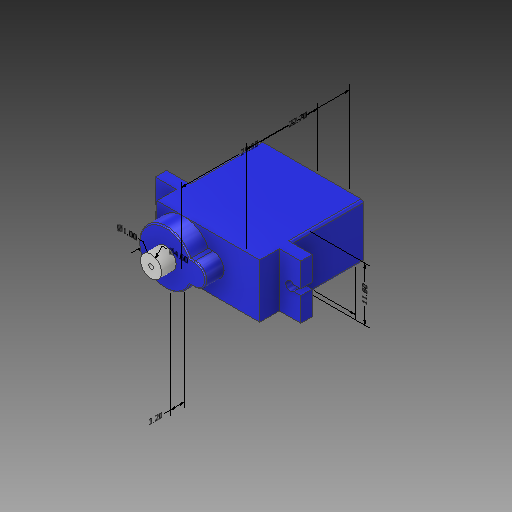
# Autodesk Inventor part: servo motor
Saved by Autodesk Inventor 2018 (Build 220112000, 112)
## iProperties
Created: 2017-05-17
Part Number: servo motor
Material: Generic
Document SubType Name: Modeling
Designer: Manh
Density: 1 g/cm^3
Appearance: Default
Author: Manh
Autodesk Inventor part; units mm, degrees
ref_plane "YZ Plane" through (0, 0, 0) normal (1, 0, 0) x (0, 1, 0)
ref_plane "XZ Plane" through (0, 0, 0) normal (0, 1, 0) x (-1, 0, 0)
ref_plane "XY Plane" through (0, 0, 0) normal (0, 0, 1) x (1, 0, 0)
sketch "Sketch1" plane through (0, 0, 0) normal (0, 0, 1) x (1, 0, 0)
  line L0 (-11.5182, 8.1773) -> (10.9818, 8.1773)
  line L1 (10.9818, 8.1773) -> (10.9818, -3.6227)
  line L2 (10.9818, -3.6227) -> (-11.5182, -3.6227)
  line L3 (-11.5182, -3.6227) -> (-11.5182, 8.1773)
  point P0 (0, 0)
  dimension "d0" = 22.5
  dimension "d1" = 11.8
  constraints: 8 end point, 2 parallel, 1 horizontal, 1 perpendicular
  measures "d0" distance of L1.end L2.end
  measures "d1" distance of L0.end L1.end
extrude "Extrusion1" add sketch "Sketch1" along normal blind 22.7
sketch "Sketch2" plane through (0, 0, 22.7) normal (0, 0, 1) x (1, 0, 0)
  arc A0 (-0.2741, 4.7773) -> (-0.2741, -0.2227) centre (-5.6182, 2.2773) ccw
  line L0 (-11.5182, 8.1773) -> (-11.5182, -3.6227) projected
  line L1 (-11.5182, -3.6227) -> (10.9818, -3.6227) projected
  line L2 (-0.2741, 4.7773) -> (0.6818, 4.7773)
  line L3 (0.6818, -0.2227) -> (-0.2741, -0.2227)
  arc A1 (0.6818, -0.2227) -> (0.6818, 4.7773) centre (0.6818, 2.2773) ccw
  line L4 (3.1818, 2.2773) -> (3.1818, 4.4746) construction
  point P0 (0, 0)
  dimension "d4" = 11.8
  dimension "d5" = 5.9
  dimension "d6" = 5
  dimension "d7" = 8.8
  dimension "d8" = 2.5
  constraints: 6 end point, 5 point on circle, 4 tangent, 2 centre point, 2 horizontal, 1 horizontal alignment, 1 vertical
  measures "d4" diameter of A0
  measures "d5" distance from line of L1 A0.centre
  measures "d6" distance of L2.end L3.start
  measures "d7" distance from line of A0.centre L4
  measures "d8" radius of A1
extrude "Extrusion2" add sketch "Sketch2" along normal blind 4 contours L2 A1 L3 A0
sketch "Sketch3" plane through (0, 0, 26.7) normal (0, 0, 1) x (1, 0, 0)
  line L0 (0.6818, 4.7773) -> (-0.2741, 4.7773) projected
  arc A0 (-0.2741, 4.7773) -> (-0.2741, -0.2227) centre (-5.6182, 2.2773) ccw projected
  line L1 (-0.2741, -0.2227) -> (0.6818, -0.2227) projected
  arc A1 (0.6818, -0.2227) -> (0.6818, 4.7773) centre (0.6818, 2.2773) ccw projected
  circle A2 centre (-5.6182, 2.2773) radius 2.3
  point P0 (0, 0)
  dimension "d11" = 4.6
  constraints: 1 centre point, 1 coincident
  measures "d11" diameter of A2
extrude "Extrusion3" add sketch "Sketch3" along normal blind 3.2 contours A2
ref_plane "Work Plane1" through (0, 0, 18.4) normal (0, 0, -1) x (-1, 0, 0)
sketch "Sketch4" plane through (0, 0, 18.4) normal (0, 0, -1) x (-1, 0, 0)
  line L0 (11.5182, 8.1773) -> (-10.9818, 8.1773) projected
  line L1 (-10.9818, 8.1773) -> (-10.9818, -3.6227) projected
  line L2 (-10.9818, -3.6227) -> (11.5182, -3.6227) projected
  line L3 (11.5182, -3.6227) -> (11.5182, 8.1773) projected
  line L4 (11.5182, 8.1773) -> (16.2182, 8.1773)
  line L5 (16.2182, 8.1773) -> (16.2182, -3.6227)
  line L6 (16.2182, -3.6227) -> (11.5182, -3.6227)
  line L7 (11.5182, -3.6227) -> (11.5182, 8.1773)
  line L8 (-10.9818, 8.1773) -> (-15.6818, 8.1773)
  line L9 (-15.6818, 8.1773) -> (-15.6818, -3.6227)
  line L10 (-15.6818, -3.6227) -> (-10.9818, -3.6227)
  line L11 (-10.9818, -3.6227) -> (-10.9818, 8.1773)
  arc A0 (14.6782, 2.9273) -> (14.6782, 1.6273) centre (13.9182, 2.2773) ccw
  arc A1 (-14.1417, 1.6273) -> (-14.1417, 2.9273) centre (-13.3818, 2.2773) ccw
  line L12 (-14.1417, 2.9273) -> (-15.6818, 2.9273)
  line L13 (-14.1417, 1.6273) -> (-15.6818, 1.6273)
  line L14 (16.2182, 2.9273) -> (14.6782, 2.9273)
  line L15 (16.2182, 1.6273) -> (14.6782, 1.6273)
  point P0 (0, 0)
  dimension "d15" = 4.7
  dimension "d16" = 4.7
  dimension "d17" = 5.9
  dimension "d18" = 5.9
  dimension "d19" = 2
  dimension "d20" = 2
  dimension "d23" = 2.3
  dimension "d24" = 2.3
  dimension "d25" = 1.3
  dimension "d26" = 1.3
  dimension "d27" = 0.65
  dimension "d28" = 0.65
  constraints: 24 end point, 6 horizontal, 5 parallel, 4 point on circle, 4 point on line, 2 centre point, 2 perpendicular, 1 horizontal alignment
  measures "d15" distance of L0.start L4.end
  measures "d16" distance of L0.end L8.end
  measures "d17" distance from line of L0 A0.centre
  measures "d18" distance from line of A1.centre L8
  measures "d19" diameter of A0
  measures "d20" diameter of A1
  measures "d23" distance from line of L9 A1.centre
  measures "d24" distance from line of L5 A0.centre
  measures "d25" distance between parallel lines of L13 L12
  measures "d26" distance between parallel lines of L15 L14
  measures "d27" distance from line of A0.centre L14
  measures "d28" distance from line of A1.centre L13
extrude "Extrusion4" add sketch "Sketch4" along normal blind 2.5 contours L4 L5 L14 A0 L15 L6 L3 | L1 L10 L9 L13 A1 L12 L8
sketch "Sketch5" plane through (-11.5182, -3.6227, 0) normal (-1, 0, 0) x (0, 0, 1)
  line L0 (5.7, 7.7) -> (4.5, 7.7)
  line L1 (4.5, 7.7) -> (4.5, 4.1)
  line L2 (4.5, 4.1) -> (5.7, 4.1)
  line L3 (5.7, 4.1) -> (5.7, 7.7)
  line L4 (0, 0) -> (0, 11.8) projected
  line L5 (0, 5.9) -> (2.0483, 5.9) construction
  point P0 (0, 3.6227)
  dimension "d31" = 1.2
  dimension "d32" = 3.6
  dimension "d33" = 4.5
  constraints: 10 end point, 2 parallel, 1 horizontal, 1 midpoint, 1 perpendicular, 1 other
  measures "d31" distance of L0.start L0.end
  measures "d32" distance of L2.end L0.start
  measures "d33" distance between parallel lines of L4 L1
fillet "Fillet1" radius 0.25 4 edges at (-11.5182, 2.2773, 26.7) (0.2038, 4.7773, 26.7) (0.2038, -0.2227, 26.7) (3.1818, 2.2773, 26.7)
sketch "Sketch6" plane through (-11.5182, -3.6227, 0) normal (-1, 0, 0) x (0, 0, 1)
  arc A0 (5.2906, 6.4417) -> (4.8906, 6.4417) centre (5.0906, 6.9) ccw
  line L0 (4.8816, 4.4457) -> (5.2851, 7.2539) construction
  line L1 (5.2906, 6.4417) -> (5.2906, 6.3583)
  line L2 (5.2906, 5.4417) -> (5.2906, 5.3583)
  arc A1 (4.8906, 5.3583) -> (5.2906, 5.3583) centre (5.0906, 4.9) ccw
  arc A2 (5.2906, 5.4417) -> (5.2906, 6.3583) centre (5.0906, 5.9) ccw
  arc A3 (4.8906, 6.3583) -> (4.8906, 5.4417) centre (5.0906, 5.9) ccw
  line L3 (5.2906, 3.9094) -> (5.0683, 6.1222) construction
  line L4 (4.8787, 7.3529) -> (4.8906, 7.2532) construction
  line L5 (4.8906, 5.3583) -> (4.8906, 5.4417)
  line L6 (4.8906, 6.3583) -> (4.8906, 6.4417)
  line L7 (0, 0) -> (0, 11.8) projected
  point P0 (0, 3.6227)
  point P1 (0, 5.9)
  dimension "d39" = 1
  dimension "d40" = 2
  dimension "d42" = 0.4
  dimension "d43" = 0.4
  dimension "d44" = 5.0906
  dimension "d45" = 0.5
  dimension "d46" = 0.5
  dimension "d47" = 0.5
  dimension "d48" = 1
  dimension "d49" = 1
  dimension "d50" = 0.2
  dimension "d51" = 0.2
  dimension "d52" = 0.2
  dimension "d53" = 0.5
  dimension "d54" = 0.2
  constraints: 14 end point, 10 point on circle, 4 centre point, 4 parallel, 2 point on line, 2 vertical alignment, 1 horizontal alignment, 1 midpoint
  measures "d39" diameter of A0
  measures "d40" distance of A0.centre A1.centre
  measures "d42" distance between parallel lines of L6 L1
  measures "d43" distance between parallel lines of L5 L2
  measures "d44" distance from line of L7 A2.centre
  measures "d45" radius of A2
  measures "d46" radius of A1
  measures "d47" radius of A0
  measures "d48" distance of A0.centre A2.centre
  measures "d49" distance of A1.centre A2.centre
  measures "d50" distance from line of L1 A0.centre
  measures "d51" distance from line of A2.centre L2
  measures "d52" distance from line of A2.centre L5
  measures "d53" radius of A3
  measures "d54" distance from line of L6 A2.centre
sketch "Sketch7" plane through (-5.6182, 2.2773, 29.9) normal (0, 0, 1) x (1, 0, 0)
  circle A0 centre (0, 0) radius 0.5
  point P0 (5.6182, -2.2773)
  dimension "d55" = 1
  constraints: 1 centre point
  measures "d55" diameter of A0
extrude "Extrusion6" cut sketch "Sketch7" against normal blind 3
fillet "Fillet2" radius 0.5 4 edges at (10.9818, 8.1773, 7.95) (-11.5182, 8.1773, 7.95) (-11.5182, -3.6227, 7.95) (10.9818, -3.6227, 7.95)
sketch "Boceto8" plane through (-5.6182, -3.6227, 22.7) normal (0, -1, 0) x (1, 0, 0)
  line L0 (-10.6, -6.8) -> (-5.4, -6.8) projected
  line L1 (-10.6, -6.8) -> (21.3, -6.8)
  line L2 (21.3, -6.8) -> (21.3, -9.8)
  line L3 (21.3, -9.8) -> (-10.6, -9.8)
  line L4 (-10.6, -9.8) -> (-10.6, -6.8)
  line L5 (-5.9, -6.8) -> (-5.9, -22.7) projected
  line L6 (16.6, -22.7) -> (16.6, -6.8) projected
  line L7 (-5.9, -6.8) -> (-5.9, -9.8)
  line L8 (16.6, -6.8) -> (16.6, -22.7) projected
  line L9 (16.6, -6.8) -> (16.6, -9.8)
  point P0 (5.6182, -22.7)
  dimension "d82" = 3
  constraints: 12 end point, 4 point on line, 2 parallel, 1 horizontal, 1 perpendicular
  measures "d82" distance of L1.end L2.end
extrude "Extrusión7" add sketch "Boceto8" against normal blind 11.8 separate body contours L0 L5 L3 L4 | L1 L2 L3 L6
sketch "Boceto9" plane through (-5.6182, -3.6227, 22.7) normal (0, -1, 0) x (1, 0, 0)
  line L0 (-10.6, -9.8) -> (-10.6, -6.8) projected
  line L1 (21.3, -6.8) -> (16.1, -6.8) projected
  line L2 (-10.6, -9.8) -> (21.3, -9.8)
  line L3 (21.3, -9.8) -> (21.3, -6.8)
  line L4 (21.3, -6.8) -> (-10.6, -6.8)
  line L5 (-10.6, -6.8) -> (-10.6, -9.8)
  point P0 (5.6182, -22.7)
  constraints: 8 end point, 2 parallel, 1 horizontal, 1 perpendicular
extrude "Extrusión8" add sketch "Boceto9" along normal blind 3 bodies 2
sketch "Boceto10" plane through (10.9818, 8.1773, 15.9) normal (0, 0, 1) x (1, 0, 0)
  arc A0 (-25.6599, -6.55) -> (-25.6599, -5.25) centre (-24.9, -5.9) ccw projected
  arc A1 (3.1599, -5.25) -> (3.1599, -6.55) centre (2.4, -5.9) ccw projected
  circle A2 centre (-24.9, -5.9) radius 1
  circle A3 centre (2.4, -5.9) radius 1
  point P0 (-10.9818, -8.1773)
  constraints: 2 centre point, 2 coincident, 2 concentric
extrude "Extrusión9" cut sketch "Boceto10" against normal blind 3 bodies 2
sketch "Boceto11" plane through (15.6818, 8.1773, 15.9) normal (1, 0, 0) x (0, 0, -1)
  line L0 (15.9, -14.8) -> (-6.8, -14.8)
  line L1 (-6.8, -14.8) -> (-6.8, 0)
  line L2 (-6.8, 0) -> (15.9, 0)
  line L3 (15.9, 0) -> (15.9, -14.8)
  point P0 (15.9, -8.1773)
  constraints: 8 end point, 2 parallel, 1 horizontal, 1 perpendicular
extrude "Extrusión10" add sketch "Boceto11" along normal blind 3 bodies 2
fillet "Empalme3" radius 3.2 1 edges at (15.6818, 0.7773, 12.9)
sketch "Boceto12" plane through (18.6818, 8.1773, 15.9) normal (1, 0, 0) x (0, 0, -1)
  circle A0 centre (2, -5.9) radius 1
  point P0 (15.9, -8.1773)
  dimension "d92" = 2
  constraints: 1 centre point, 1 coincident, 1 other
  measures "d92" diameter of A0
extrude "Extrusión11" cut sketch "Boceto12" against normal blind 2 bodies 2
body "Solid1"
